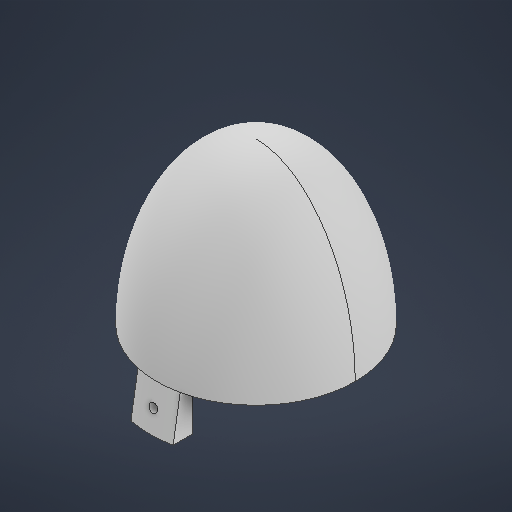
# Autodesk Inventor part: 005-001
Saved by Autodesk Inventor 2026 (Build 300175000, 175)
## iProperties
Created: 2026-04-20
Part Number: 005-001
Material: Ogólny
Document SubType Name: Modeling
Designer: Patryk Lombardo
Density: 1 g/cm^3
Appearance: Domyślna
Author: Patryk Lombardo
Autodesk Inventor part; units mm, degrees
ref_plane "YZ Plane" through (0, 0, 0) normal (1, 0, 0) x (0, 1, 0)
ref_plane "XZ Plane" through (0, 0, 0) normal (0, 1, 0) x (-1, 0, 0)
sketch "Szkic1" plane through (0, 0, 0) normal (0, 0, 1) x (1, 0, 0)
  line L0 (0, 0) -> (18.5, 0) construction
  line L1 (18.5, 0) -> (23.5, 0)
  line L2 (0, 0) -> (0, 33) construction
  line L3 (0, 33) -> (0, 38)
  ellipse E0 centre (0, 0) end of major axis (23.5, 0) minor radius 38 (23.5, 0) -> (0, 38) ccw
  ellipse E1 centre (0, 0) end of major axis (18.5, 0) minor radius 33 (18.5, 0) -> (0, 33) ccw
  dimension "d0" = 18.5
  dimension "d1" = 5
  dimension "d2" = 33
  dimension "d3" = 5
  constraints: 8 end point, 3 horizontal, 2 coincident, 2 vertical, 8 other
  measures "d0" distance of L0.start L0.end
  measures "d1" distance of L0.end L1.end
  measures "d2" distance of L0.start L2.end
  measures "d3" distance of L2.end L3.end
revolve "Obrót1" add sketch "Szkic1" angle 360 about axis through (0, 0, 0) along (0, 1, 0)
ref_plane "Płaszczyzna konstrukcyjna1" through (0, -10, 0) normal (0, -1, 0) x (1, 0, 0)
sketch "Szkic2" plane through (0, -10, 0) normal (0, -1, 0) x (1, 0, 0)
  circle A0 centre (0, 0) radius 25.122
  dimension "d6" = 50.244
  constraints: 1 centre point, 1 coincident
  measures "d6" diameter of A0
loft "Wyciągnięcie złożone1" add profiles "Szkic2" section 2 edges at (-23.5, 0, 0)
sketch "Szkic3" plane through (0, -10, 0) normal (0, -1, 0) x (1, 0, 0)
  circle A0 centre (0, 0) radius 23.5
  line L0 (0, -20) -> (0, 20) construction
  line L1 (-5, 20) -> (5, 20)
  line L2 (-5, -20) -> (5, -20)
  line L3 (5, 20) -> (5, 30)
  line L4 (5, -20) -> (5, -30)
  line L5 (-5, -20) -> (-5, -30)
  line L6 (-5, -30) -> (5, -30)
  line L7 (-5, 20) -> (-5, 30)
  line L8 (-5, 30) -> (5, 30)
  circle A1 centre (0, 0) radius 27.5
  point P0 (-5, 27.0416)
  point P1 (-5, -27.0416)
  point P2 (5, -27.0416)
  point P3 (5, 27.0416)
  dimension "d11" = 47
  dimension "d12" = 40
  dimension "d13" = 10
  dimension "d14" = 10
  dimension "d15" = 10
  dimension "d16" = 10
  dimension "d17" = 55
  constraints: 18 end point, 4 vertical, 3 coincident, 3 midpoint, 2 centre point, 2 horizontal, 2 perpendicular, 1 point on line
  measures "d11" diameter of A0
  measures "d12" distance of L0.start L0.end
  measures "d13" distance of L2.start L2.end
  measures "d14" distance of L1.start L1.end
  measures "d15" distance of L1.end L3.end
  measures "d16" distance of L2.end L4.end
  measures "d17" diameter of A1
extrude "Wyciągnięcie proste1" cut sketch "Szkic3" against normal blind 10 contours A0 L4 L2 L5 L7 L1 L3 | A0 L3 A1 L4 | A0 L5 A1 L7
sketch "Szkic4" plane through (-5, -10, -20) normal (0, 0, 1) x (1, 0, 0)
  line L0 (5, 10) -> (5, 5) construction
  circle A0 centre (5, 5) radius 1
  dimension "d20" = 5
  dimension "d21" = 2
  constraints: 2 end point, 1 centre point, 1 coincident, 1 vertical
  measures "d20" distance of L0.start L0.end
  measures "d21" diameter of A0
extrude "Wyciągnięcie proste2" cut sketch "Szkic4" along normal through all both and the other way through all
